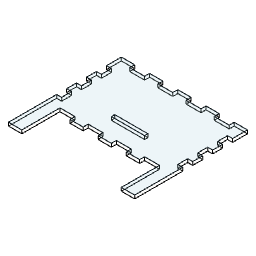
case_2_3mm (Autodesk Fusion 360 design; units mm, degrees)
Autodesk Fusion 360 part; units mm, degrees
sketch "スケッチ1" plane through (0, 0, 0) normal (0, 0, 1) x (1, 0, 0)
  line L0 (0, 0) -> (74, 0)
  line L1 (74, 0) -> (74, 46)
  line L2 (74, 46) -> (0, 46)
  line L3 (0, 46) -> (0, 0)
  dimension "d1" = 46
  dimension "d2" = 74
  constraint horizontal L0
  constraint vertical L1
  constraint horizontal L2
  constraint vertical L3
  constraint coincident L0.start L3.end
  measures "d1" distance of L0.start L2.end
  measures "d2" distance of L0.start L0.end
extrude "押し出し1" add sketch "スケッチ1" along normal blind 2
sketch "スケッチ2" plane through (0, 0, 2) normal (0, 0, 1) x (-1, 0, 0)
  line L0 (0, -46) -> (0, 0)
  line L1 (0, 0) -> (-74, 0)
  line L2 (-74, 0) -> (-74, -46)
  line L3 (-74, -46) -> (0, -46)
  line L4 (-27, -13) -> (-47, -13)
  line L5 (-47, -13) -> (-47, -15)
  line L6 (-47, -15) -> (-27, -15)
  line L7 (-27, -15) -> (-27, -13)
  dimension "d5" = 2
  dimension "d6" = 20
  dimension "d7" = 13
  dimension "d8" = 27
  constraint horizontal L4
  constraint vertical L5
  constraint horizontal L6
  constraint vertical L7
  measures "d5" distance of L4.end L5.end
  measures "d6" distance of L4.start L4.end
  measures "d7" distance of L1 L4
  measures "d8" distance of L2 L5
extrude "押し出し2" cut sketch "スケッチ2" against normal blind 2 contours L4 L5 L6 L7
sketch "スケッチ3" plane through (0, 0, 2) normal (0, 0, 1) x (-1, 0, 0)
  line L0 (-47, -13) -> (-27, -13)
  line L1 (-27, -13) -> (-27, -15)
  line L2 (-27, -15) -> (-47, -15)
  line L3 (-47, -15) -> (-47, -13)
  line L4 (0, -46) -> (0, 0)
  line L5 (0, 0) -> (-74, 0)
  line L6 (-74, 0) -> (-74, -46)
  line L7 (-74, -46) -> (0, -46)
  line L8 (-67, -46) -> (-58, -46)
  line L9 (-58, -46) -> (-58, -44)
  line L10 (-58, -44) -> (-67, -44)
  line L11 (-67, -44) -> (-67, -46)
  line L12 (-50, -46) -> (-41, -46)
  line L13 (-50, -44) -> (-50, -46)
  line L14 (-41, -44) -> (-50, -44)
  line L15 (-41, -46) -> (-41, -44)
  line L16 (-33, -46) -> (-24, -46)
  line L17 (-33, -44) -> (-33, -46)
  line L18 (-24, -44) -> (-33, -44)
  line L19 (-24, -46) -> (-24, -44)
  line L20 (-16, -46) -> (-7, -46)
  line L21 (-16, -44) -> (-16, -46)
  line L22 (-7, -44) -> (-16, -44)
  line L23 (-7, -46) -> (-7, -44)
  line L24 (-24, 0) -> (-33, 0)
  line L25 (-33, 0) -> (-33, -2)
  line L26 (-58, 0) -> (-67, 0)
  line L27 (-50, 0) -> (-50, -2)
  line L28 (-50, -2) -> (-41, -2)
  line L29 (-7, -2) -> (-7, 0)
  line L30 (-7, 0) -> (-16, 0)
  line L31 (-16, 0) -> (-16, -2)
  line L32 (-33, -2) -> (-24, -2)
  line L33 (-67, 0) -> (-67, -2)
  line L34 (-41, -2) -> (-41, 0)
  line L35 (-16, -2) -> (-7, -2)
  line L36 (-24, -2) -> (-24, 0)
  line L37 (-41, 0) -> (-50, 0)
  line L38 (-67, -2) -> (-58, -2)
  line L39 (-58, -2) -> (-58, 0)
  line L40 (0, -38) -> (-2, -38)
  line L41 (-2, -38) -> (-2, -32)
  line L42 (-2, -32) -> (0, -32)
  line L43 (0, -32) -> (0, -38)
  line L44 (-2, -20) -> (0, -20)
  line L45 (-2, -26) -> (-2, -20)
  line L46 (0, -26) -> (-2, -26)
  line L47 (0, -20) -> (0, -26)
  line L48 (-2, -8) -> (0, -8)
  line L49 (-2, -14) -> (-2, -8)
  line L50 (0, -14) -> (-2, -14)
  line L51 (0, -8) -> (0, -14)
  line L52 (-74, -20) -> (-72, -20)
  line L53 (-72, -8) -> (-72, -14)
  line L54 (-74, -8) -> (-72, -8)
  line L55 (-72, -14) -> (-74, -14)
  line L56 (-74, -38) -> (-74, -32)
  line L57 (-72, -32) -> (-72, -38)
  line L58 (-72, -26) -> (-74, -26)
  line L59 (-74, -32) -> (-72, -32)
  line L60 (-74, -14) -> (-74, -8)
  line L61 (-72, -20) -> (-72, -26)
  line L62 (-74, -26) -> (-74, -20)
  line L63 (-72, -38) -> (-74, -38)
  dimension "d11" = 9
  dimension "d12" = 2
  dimension "d13" = 7
  dimension "d16" = 17
  dimension "d17" = 0
  dimension "d20" = 0
  dimension "d21" = 44
  dimension "d22" = 6
  dimension "d23" = 2
  dimension "d24" = 8
  dimension "d27" = 0
  dimension "d28" = 12
  dimension "d31" = -72
  dimension "d32" = 0
  constraint horizontal L8
  constraint vertical L9
  constraint horizontal L10
  constraint vertical L11
  constraint coincident L7 L8.start
  constraint horizontal L40
  constraint vertical L41
  constraint horizontal L42
  constraint vertical L43
  constraint coincident L4 L40.start
  measures "d11" distance of L8.start L8.end
  measures "d12" distance of L8.start L10.end
  measures "d13" distance of L6 L11
  measures "d22" distance of L40.start L42.end
  measures "d23" distance of L40.start L40.end
  measures "d24" distance of L7 L40
extrude "押し出し3" cut sketch "スケッチ3" against normal blind 2 contours L4 L40 L41 L42 L43 | L7 L20 L21 L22 L23 | L4 L44 L45 L46 L47 | L7 L16 L17 L18 L19 | L4 L48 L49 L50 L51 | L7 L12 L13 L14 L15 | L7 L8 L9 L10 L11 | L5 L29 L30 L31 L35 | L5 L24 L25 L32 L36 | L6 L56 L57 L59 L63 | L5 L27 L28 L34 L37 | L6 L52 L58 L61 L62 | L5 L26 L33 L38 L39 | L6 L53 L54 L55 L60
sketch "スケッチ4" plane through (0, 0, 2) normal (0, 0, 1) x (-1, 0, 0)
  line L0 (-50, -2) -> (-50, 0)
  line L1 (-50, 0) -> (-58, 0)
  line L2 (-58, 0) -> (-58, -2)
  line L3 (-58, -2) -> (-67, -2)
  line L4 (-67, -2) -> (-67, 0)
  line L5 (-67, 0) -> (-74, 0)
  line L6 (-74, 0) -> (-74, -8)
  line L7 (-74, -8) -> (-72, -8)
  line L8 (-72, -8) -> (-72, -14)
  line L9 (-72, -14) -> (-74, -14)
  line L10 (-74, -14) -> (-74, -20)
  line L11 (-74, -20) -> (-72, -20)
  line L12 (-72, -20) -> (-72, -26)
  line L13 (-72, -26) -> (-74, -26)
  line L14 (-74, -26) -> (-74, -32)
  line L15 (-74, -32) -> (-72, -32)
  line L16 (-72, -32) -> (-72, -38)
  line L17 (-72, -38) -> (-74, -38)
  line L18 (-74, -38) -> (-74, -46)
  line L19 (-74, -46) -> (-67, -46)
  line L20 (-67, -46) -> (-67, -44)
  line L21 (-67, -44) -> (-58, -44)
  line L22 (-58, -44) -> (-58, -46)
  line L23 (-58, -46) -> (-50, -46)
  line L24 (-50, -46) -> (-50, -44)
  line L25 (-50, -44) -> (-41, -44)
  line L26 (-41, -44) -> (-41, -46)
  line L27 (-41, -46) -> (-33, -46)
  line L28 (-33, -46) -> (-33, -44)
  line L29 (-33, -44) -> (-24, -44)
  line L30 (-24, -44) -> (-24, -46)
  line L31 (-24, -46) -> (-16, -46)
  line L32 (-16, -46) -> (-16, -44)
  line L33 (-16, -44) -> (-7, -44)
  line L34 (-7, -44) -> (-7, -46)
  line L35 (-7, -46) -> (0, -46)
  line L36 (0, -46) -> (0, -38)
  line L37 (0, -38) -> (-2, -38)
  line L38 (-2, -38) -> (-2, -32)
  line L39 (-2, -32) -> (0, -32)
  line L40 (0, -32) -> (0, -26)
  line L41 (0, -26) -> (-2, -26)
  line L42 (-2, -26) -> (-2, -20)
  line L43 (-2, -20) -> (0, -20)
  line L44 (0, -20) -> (0, -14)
  line L45 (0, -14) -> (-2, -14)
  line L46 (-2, -14) -> (-2, -8)
  line L47 (-2, -8) -> (0, -8)
  line L48 (0, -8) -> (0, 0)
  line L49 (0, 0) -> (-7, 0)
  line L50 (-7, 0) -> (-7, -2)
  line L51 (-7, -2) -> (-16, -2)
  line L52 (-16, -2) -> (-16, 0)
  line L53 (-16, 0) -> (-24, 0)
  line L54 (-24, 0) -> (-24, -2)
  line L55 (-24, -2) -> (-33, -2)
  line L56 (-33, -2) -> (-33, 0)
  line L57 (-33, 0) -> (-41, 0)
  line L58 (-41, 0) -> (-41, -2)
  line L59 (-41, -2) -> (-50, -2)
  line L60 (-47, -13) -> (-27, -13)
  line L61 (-27, -13) -> (-27, -15)
  line L62 (-27, -15) -> (-47, -15)
  line L63 (-47, -15) -> (-47, -13)
  line L64 (0, 0) -> (0, 20)
  line L65 (0, 20) -> (-7, 20)
  line L66 (-7, 20) -> (-7, 0)
  line L67 (-74, 0) -> (-74, 20)
  line L68 (-74, 20) -> (-67, 20)
  line L69 (-67, 20) -> (-67, 0)
  constraint vertical L64
  constraint horizontal L65
  constraint vertical L66
  constraint coincident L49.end L50.start
  constraint vertical L67
  constraint horizontal L68
  constraint vertical L69
  constraint coincident L4.end L5.start
extrude "押し出し4" add sketch "スケッチ4" against normal blind 2 contours L5 L67 L68 L69 | L49 L64 L65 L66
sketch "スケッチ5" plane through (0, 0, 2) normal (0, 0, 1) x (-1, 0, 0)
  line L0 (-50, -2) -> (-50, 0)
  line L1 (-50, 0) -> (-58, 0)
  line L2 (-58, 0) -> (-58, -2)
  line L3 (-58, -2) -> (-67, -2)
  line L4 (-67, -2) -> (-67, 20)
  line L5 (-67, 20) -> (-74, 20)
  line L6 (-74, 20) -> (-74, -8)
  line L7 (-74, -8) -> (-72, -8)
  line L8 (-72, -8) -> (-72, -14)
  line L9 (-72, -14) -> (-74, -14)
  line L10 (-74, -14) -> (-74, -20)
  line L11 (-74, -20) -> (-72, -20)
  line L12 (-72, -20) -> (-72, -26)
  line L13 (-72, -26) -> (-74, -26)
  line L14 (-74, -26) -> (-74, -32)
  line L15 (-74, -32) -> (-72, -32)
  line L16 (-72, -32) -> (-72, -38)
  line L17 (-72, -38) -> (-74, -38)
  line L18 (-74, -38) -> (-74, -46)
  line L19 (-74, -46) -> (-67, -46)
  line L20 (-67, -46) -> (-67, -44)
  line L21 (-67, -44) -> (-58, -44)
  line L22 (-58, -44) -> (-58, -46)
  line L23 (-58, -46) -> (-50, -46)
  line L24 (-50, -46) -> (-50, -44)
  line L25 (-50, -44) -> (-41, -44)
  line L26 (-41, -44) -> (-41, -46)
  line L27 (-41, -46) -> (-33, -46)
  line L28 (-33, -46) -> (-33, -44)
  line L29 (-33, -44) -> (-24, -44)
  line L30 (-24, -44) -> (-24, -46)
  line L31 (-24, -46) -> (-16, -46)
  line L32 (-16, -46) -> (-16, -44)
  line L33 (-16, -44) -> (-7, -44)
  line L34 (-7, -44) -> (-7, -46)
  line L35 (-7, -46) -> (0, -46)
  line L36 (0, -46) -> (0, -38)
  line L37 (0, -38) -> (-2, -38)
  line L38 (-2, -38) -> (-2, -32)
  line L39 (-2, -32) -> (0, -32)
  line L40 (0, -32) -> (0, -26)
  line L41 (0, -26) -> (-2, -26)
  line L42 (-2, -26) -> (-2, -20)
  line L43 (-2, -20) -> (0, -20)
  line L44 (0, -20) -> (0, -14)
  line L45 (0, -14) -> (-2, -14)
  line L46 (-2, -14) -> (-2, -8)
  line L47 (-2, -8) -> (0, -8)
  line L48 (0, -8) -> (0, 20)
  line L49 (0, 20) -> (-7, 20)
  line L50 (-7, 20) -> (-7, -2)
  line L51 (-7, -2) -> (-16, -2)
  line L52 (-16, -2) -> (-16, 0)
  line L53 (-16, 0) -> (-24, 0)
  line L54 (-24, 0) -> (-24, -2)
  line L55 (-24, -2) -> (-33, -2)
  line L56 (-33, -2) -> (-33, 0)
  line L57 (-33, 0) -> (-41, 0)
  line L58 (-41, 0) -> (-41, -2)
  line L59 (-41, -2) -> (-50, -2)
  line L60 (-47, -13) -> (-27, -13)
  line L61 (-27, -13) -> (-27, -15)
  line L62 (-27, -15) -> (-47, -15)
  line L63 (-47, -15) -> (-47, -13)
  line L64 (0, -47) -> (-7, -47)
  line L65 (-7, -47) -> (-7, -46)
  line L66 (-7, -46) -> (0, -46)
  line L67 (0, -46) -> (0, -47)
  line L68 (-16, -46) -> (-24, -46)
  line L69 (-24, -46) -> (-24, -47)
  line L70 (-24, -47) -> (-16, -47)
  line L71 (-16, -47) -> (-16, -46)
  line L72 (-33, -46) -> (-41, -46)
  line L73 (-41, -46) -> (-41, -47)
  line L74 (-41, -47) -> (-33, -47)
  line L75 (-33, -47) -> (-33, -46)
  line L76 (-50, -46) -> (-58, -46)
  line L77 (-58, -46) -> (-58, -47)
  line L78 (-58, -47) -> (-50, -47)
  line L79 (-50, -47) -> (-50, -46)
  line L80 (-67, -46) -> (-75, -46)
  line L81 (-75, -46) -> (-75, -47)
  line L82 (-75, -47) -> (-67, -47)
  line L83 (-67, -47) -> (-67, -46)
  line L84 (-75, -46) -> (-74, -46)
  line L85 (-74, -46) -> (-74, -38)
  line L86 (-74, -38) -> (-75, -38)
  line L87 (-75, -38) -> (-75, -46)
  line L88 (-75, -32) -> (-74, -32)
  line L89 (-74, -32) -> (-74, -26)
  line L90 (-74, -26) -> (-75, -26)
  line L91 (-75, -26) -> (-75, -32)
  line L92 (-75, -20) -> (-74, -20)
  line L93 (-74, -20) -> (-74, -14)
  line L94 (-74, -14) -> (-75, -14)
  line L95 (-75, -14) -> (-75, -20)
  line L96 (-75, -8) -> (-74, -8)
  line L97 (-74, -8) -> (-74, 20)
  line L98 (-74, 20) -> (-75, 20)
  line L99 (-75, 20) -> (-75, -8)
  line L100 (-75, 21) -> (-67, 21)
  line L101 (-67, 21) -> (-67, 20)
  line L102 (-67, 20) -> (-75, 20)
  line L103 (-75, 20) -> (-75, 21)
  line L104 (-58, 0) -> (-50, 0)
  line L105 (-50, 0) -> (-50, 1)
  line L106 (-50, 1) -> (-58, 1)
  line L107 (-58, 1) -> (-58, 0)
  line L108 (-41, 0) -> (-33, 0)
  line L109 (-33, 0) -> (-33, 1)
  line L110 (-33, 1) -> (-41, 1)
  line L111 (-41, 1) -> (-41, 0)
  line L112 (-24, 0) -> (-16, 0)
  line L113 (-16, 0) -> (-16, 1)
  line L114 (-16, 1) -> (-24, 1)
  line L115 (-24, 1) -> (-24, 0)
  line L116 (-7, 20) -> (1, 20)
  line L117 (1, 20) -> (1, 21)
  line L118 (1, 21) -> (-7, 21)
  line L119 (-7, 21) -> (-7, 20)
  line L120 (1, 20) -> (0, 20)
  line L121 (0, 20) -> (0, -8)
  line L122 (0, -8) -> (1, -8)
  line L123 (1, -8) -> (1, 20)
  line L124 (1, -14) -> (0, -14)
  line L125 (0, -14) -> (0, -20)
  line L126 (0, -20) -> (1, -20)
  line L127 (1, -20) -> (1, -14)
  line L128 (1, -26) -> (0, -26)
  line L129 (0, -26) -> (0, -32)
  line L130 (0, -32) -> (1, -32)
  line L131 (1, -32) -> (1, -26)
  line L132 (0, -38) -> (1, -38)
  line L133 (1, -38) -> (1, -47)
  line L134 (1, -47) -> (0, -47)
  line L135 (0, -47) -> (0, -38)
  constraint horizontal L64
  constraint vertical L65
  constraint horizontal L66
  constraint vertical L67
  constraint coincident L34.end L35.start
  constraint horizontal L68
  constraint vertical L69
  constraint horizontal L70
  constraint vertical L71
  constraint coincident L31.end L32.start
  constraint horizontal L72
  constraint vertical L73
  constraint horizontal L74
  constraint vertical L75
  constraint coincident L27.end L28.start
  constraint horizontal L76
  constraint vertical L77
  constraint horizontal L78
  constraint vertical L79
  constraint coincident L23.end L24.start
  constraint horizontal L80
  constraint vertical L81
  constraint horizontal L82
  constraint vertical L83
  constraint coincident L19.end L20.start
  constraint horizontal L84
  constraint vertical L85
  constraint horizontal L86
  constraint vertical L87
  constraint coincident L17.end L18.start
  constraint horizontal L88
  constraint vertical L89
  constraint horizontal L90
  constraint vertical L91
  constraint coincident L13.end L14.start
  constraint horizontal L92
  constraint vertical L93
  constraint horizontal L94
  constraint vertical L95
  constraint coincident L9.end L10.start
  constraint horizontal L96
  constraint vertical L97
  constraint horizontal L98
  constraint vertical L99
  constraint coincident L5.end L6.start
  constraint horizontal L100
  constraint vertical L101
  constraint horizontal L102
  constraint vertical L103
  constraint coincident L4.end L5.start
  constraint horizontal L104
  constraint vertical L105
  constraint horizontal L106
  constraint vertical L107
  constraint coincident L1.end L2.start
  constraint horizontal L108
  constraint vertical L109
  constraint horizontal L110
  constraint vertical L111
  constraint coincident L57.end L58.start
  constraint horizontal L112
  constraint vertical L113
  constraint horizontal L114
  constraint vertical L115
  constraint coincident L53.end L54.start
  constraint horizontal L116
  constraint vertical L117
  constraint horizontal L118
  constraint vertical L119
  constraint coincident L49.end L50.start
  constraint horizontal L120
  constraint vertical L121
  constraint horizontal L122
  constraint vertical L123
  constraint coincident L47.end L48.start
  constraint horizontal L124
  constraint vertical L125
  constraint horizontal L126
  constraint vertical L127
  constraint coincident L43.end L44.start
  constraint horizontal L128
  constraint vertical L129
  constraint horizontal L130
  constraint vertical L131
  constraint coincident L39.end L40.start
  constraint horizontal L132
  constraint vertical L133
  constraint horizontal L134
  constraint vertical L135
  constraint coincident L36.end L37.start
extrude "押し出し5" add sketch "スケッチ5" against normal blind 2 contours L1 L104 L105 L106 L107 | L57 L108 L109 L110 L111 | L5 L98 L100 L101 L102 L103 | L6 L96 L97 L98 L99 L102 | L53 L112 L113 L114 L115 | L10 L92 L93 L94 L95 | L49 L116 L117 L118 L119 L120 | L48 L116 L120 L121 L122 L123 | L14 L88 L89 L90 L91 | L44 L124 L125 L126 L127 | L18 L80 L84 L85 L86 L87 | L19 L80 L81 L82 L83 L84 | L40 L128 L129 L130 L131 | L23 L76 L77 L78 L79 | L36 L67 L132 L133 L134 L135 | L35 L64 L65 L66 L67 L135 | L27 L72 L73 L74 L75 | L31 L68 L69 L70 L71
sketch "スケッチ6" plane through (0, 0, 2) normal (0, 0, 1) x (-1, 0, 0)
  line L0 (-50, -2) -> (-50, 1)
  line L1 (-50, 1) -> (-58, 1)
  line L2 (-58, 1) -> (-58, -2)
  line L3 (-58, -2) -> (-67, -2)
  line L4 (-67, -2) -> (-67, 21)
  line L5 (-67, 21) -> (-75, 21)
  line L6 (-75, 21) -> (-75, -8)
  line L7 (-75, -8) -> (-72, -8)
  line L8 (-72, -8) -> (-72, -14)
  line L9 (-72, -14) -> (-75, -14)
  line L10 (-75, -14) -> (-75, -20)
  line L11 (-75, -20) -> (-72, -20)
  line L12 (-72, -20) -> (-72, -26)
  line L13 (-72, -26) -> (-75, -26)
  line L14 (-75, -26) -> (-75, -32)
  line L15 (-75, -32) -> (-72, -32)
  line L16 (-72, -32) -> (-72, -38)
  line L17 (-72, -38) -> (-75, -38)
  line L18 (-75, -38) -> (-75, -47)
  line L19 (-75, -47) -> (-67, -47)
  line L20 (-67, -47) -> (-67, -44)
  line L21 (-67, -44) -> (-58, -44)
  line L22 (-58, -44) -> (-58, -47)
  line L23 (-58, -47) -> (-50, -47)
  line L24 (-50, -47) -> (-50, -44)
  line L25 (-50, -44) -> (-41, -44)
  line L26 (-41, -44) -> (-41, -47)
  line L27 (-41, -47) -> (-33, -47)
  line L28 (-33, -47) -> (-33, -44)
  line L29 (-33, -44) -> (-24, -44)
  line L30 (-24, -44) -> (-24, -47)
  line L31 (-24, -47) -> (-16, -47)
  line L32 (-16, -47) -> (-16, -44)
  line L33 (-16, -44) -> (-7, -44)
  line L34 (-7, -44) -> (-7, -47)
  line L35 (-7, -47) -> (1, -47)
  line L36 (1, -47) -> (1, -38)
  line L37 (1, -38) -> (-2, -38)
  line L38 (-2, -38) -> (-2, -32)
  line L39 (-2, -32) -> (1, -32)
  line L40 (1, -32) -> (1, -26)
  line L41 (1, -26) -> (-2, -26)
  line L42 (-2, -26) -> (-2, -20)
  line L43 (-2, -20) -> (1, -20)
  line L44 (1, -20) -> (1, -14)
  line L45 (1, -14) -> (-2, -14)
  line L46 (-2, -14) -> (-2, -8)
  line L47 (-2, -8) -> (1, -8)
  line L48 (1, -8) -> (1, 21)
  line L49 (1, 21) -> (-7, 21)
  line L50 (-7, 21) -> (-7, -2)
  line L51 (-7, -2) -> (-16, -2)
  line L52 (-16, -2) -> (-16, 1)
  line L53 (-16, 1) -> (-24, 1)
  line L54 (-24, 1) -> (-24, -2)
  line L55 (-24, -2) -> (-33, -2)
  line L56 (-33, -2) -> (-33, 1)
  line L57 (-33, 1) -> (-41, 1)
  line L58 (-41, 1) -> (-41, -2)
  line L59 (-41, -2) -> (-50, -2)
  line L60 (-47, -13) -> (-27, -13)
  line L61 (-27, -13) -> (-27, -15)
  line L62 (-27, -15) -> (-47, -15)
  line L63 (-47, -15) -> (-47, -13)
